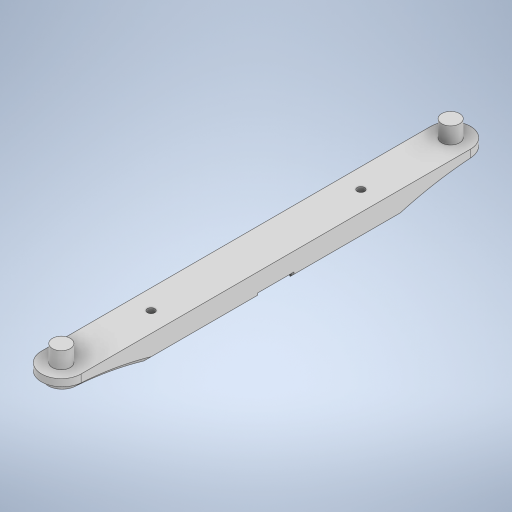
# Autodesk Inventor part: gripper_mechanism
Saved by Autodesk Inventor 2023 (Build 270158000, 158)
## iProperties
Created: 2024-07-03
Part Number: gripper_mechanism
Material: Generic
Document SubType Name: Modeling
Designer: Swoby
Density: 1 g/cm^3
Appearance: Default
Author: Swoby
Autodesk Inventor part; units mm, degrees
ref_plane "YZ Plane" through (0, 0, 0) normal (1, 0, 0) x (0, 1, 0)
ref_plane "XZ Plane" through (0, 0, 0) normal (0, 1, 0) x (-1, 0, 0)
ref_plane "XY Plane" through (0, 0, 0) normal (0, 0, 1) x (1, 0, 0)
sketch "Sketch1" plane through (0, 0, 0) normal (0, 1, 0) x (-1, 0, 0)
  circle A0 centre (0, 29.5) radius 1.5
  circle A1 centre (0, -29.5) radius 1.5
  line L0 (0, 29.5) -> (0, -29.5) construction
  circle A2 centre (0, 29.5) radius 3
  circle A3 centre (0, -29.5) radius 3
  line L1 (3, 29.5) -> (3, -29.5)
  line L2 (-3, 29.5) -> (-3, -29.5)
  point P0 (0, 0)
  dimension "d0" = 59
  dimension "d1" = 29.5
  dimension "d2" = 3
  dimension "d3" = 3
  dimension "d4" = 6
  dimension "d5" = 6
  constraints: 6 end point, 4 centre point, 4 point on circle, 4 tangent, 2 coincident, 1 midpoint, 1 vertical
  measures "d0" distance of L0.end L0.start
  measures "d1" distance of L0.start point (0, 0)
  measures "d2" diameter of A0
  measures "d3" diameter of A1
  measures "d4" diameter of A2
  measures "d5" diameter of A3
extrude "Extrusion1" add sketch "Sketch1" along normal blind 4.05
sketch "Sketch2" plane through (0, 0, 0) normal (0, -1, 0) x (1, 0, 0)
  circle A0 centre (0, 0) radius 3.75
  dimension "d8" = 7.5
  constraints: 1 centre point, 1 coincident
  measures "d8" diameter of A0
extrude "Extrusion2" cut sketch "Sketch2" against normal blind 1.3
sketch "Sketch3" plane through (0, 0, 0) normal (0, -1, 0) x (1, 0, 0)
  circle A0 centre (0, 15.9) radius 0.55
  arc A1 (3, 2.25) -> (-3, 2.25) centre (0, 0) ccw projected
  line L0 (3, 29.5) -> (3, 2.25) projected
  arc A2 (3, 29.5) -> (-3, 29.5) centre (0, 29.5) ccw projected
  line L1 (-3, 2.25) -> (-3, 29.5) projected
  circle A3 centre (0, 29.5) radius 1.5 projected
  arc A4 (-3, -2.25) -> (3, -2.25) centre (0, 0) ccw projected
  line L2 (-3, -29.5) -> (-3, -2.25) projected
  arc A5 (-3, -29.5) -> (3, -29.5) centre (0, -29.5) ccw projected
  line L3 (3, -2.25) -> (3, -29.5) projected
  circle A6 centre (0, -29.5) radius 1.5 projected
  arc A7 (3, 29.5) -> (-3, 29.5) centre (0, 29.5) ccw projected
  line L4 (0, 29.5) -> (0, -29.5)
  circle A8 centre (0, -15.9) radius 0.55
  dimension "d11" = 1.1
  dimension "d12" = 15.9
  dimension "d40" = 1.1
  dimension "d41" = 15.9
  constraints: 2 centre point, 2 end point, 2 point on line, 1 midpoint, 1 vertical
  measures "d11" diameter of A0
  measures "d12" distance of point (0, 0) A0.centre
  measures "d40" diameter of A8
  measures "d41" distance of point (0, 0) A8.centre
extrude "Extrusion3" cut sketch "Sketch3" against normal blind 4.05 contours A0 L4 | L4 A0 | A8 L4 | L4 A8
sketch "Sketch4" plane through (3, 0, -29.5) normal (1, 0, 0) x (0, 0, -1)
  line L0 (-59, 0) -> (-31.75, 0) projected
  line L1 (-62, 0) -> (-62, 4.05) projected
  arc A0 (-48.5, 0) -> (-62, 2) centre (-62.5089, -47.9974) ccw
  line L2 (-62, 2) -> (-62, 0)
  line L3 (-48.5, 0) -> (-62, 0)
  line L4 (3, 2) -> (3, 0)
  line L5 (3, 0) -> (-10.5, 0)
  arc A1 (3, 2) -> (-10.5, 0) centre (3.5089, -47.9974) ccw
  line L6 (3, 0) -> (3, 4.05) projected
  line L7 (-27.25, 1.3) -> (-27.25, 0) projected
  line L8 (-27.25, 0) -> (0, 0) projected
  line L9 (0, 0) -> (0, 4.05) projected
  line L10 (-59, 4.05) -> (0, 4.05) projected
  line L11 (-59, 0) -> (-59, 4.05) projected
  line L12 (-59, 0) -> (-31.75, 0) projected
  line L13 (-31.75, 0) -> (-31.75, 1.3) projected
  line L14 (-31.75, 1.3) -> (-27.25, 1.3) projected
  point P0 (-29.5, 1.3)
  dimension "d18" = 38
  dimension "d19" = 19
  dimension "d20" = 2
  dimension "d21" = 2
  dimension "d22" = 50
  dimension "d23" = 50
  constraints: 8 end point, 5 point on line, 4 point on circle, 2 centre point, 2 collinear, 1 midpoint, 1 perpendicular
  measures "d18" distance of L5.end L3.start
  measures "d19" horizontal distance of L5.end point (-29.5, 1.3)
  measures "d20" distance of L1.start L2.start
  measures "d21" distance of L4.end L4.start
  measures "d22" radius of A0
  measures "d23" radius of A1
extrude "Extrusion4" cut sketch "Sketch4" against normal through all contours L11 A0 L0 | L3 L1 A0 L11 | L9 L5 A1 | A1 L4 L5 L9
chamfer "Chamfer2" distance 1 angle 45 12 edges at (3, 1.2205, 24.1997) (1.9501, 1.9875, 31.7797) (-1.9483, 1.9875, 31.7813) (-3, 1.2205, 24.1997) (3, 0, 10.625) (-3, 0, 10.625) (1.9483, 1.9875, -31.7813) (-1.9501, 1.9875, -31.7797) (-3, 1.2205, -24.1997) (3, 1.2205, -24.1997) (-3, 0, -10.625) (3, 0, -10.625)
chamfer "Chamfer3" distance 0.5 angle 45 4 edges at (-3, 1.15, 2.25) (3, 1.15, 2.25) (-3, 1.15, -2.25) (3, 1.15, -2.25)
sketch "Sketch5" plane through (0, 4.05, 0) normal (0, 1, 0) x (1, 0, 0)
  circle A0 centre (0, -29.5) radius 1.5 projected
  circle A1 centre (0, 29.5) radius 1.5 projected
  point P0 (0, 0)
extrude "Extrusion5" add sketch "Sketch5" against normal blind 2.3
sketch "Sketch6" plane through (0, 1.75, 29.5) normal (0, -1, 0) x (1, 0, 0)
  circle A0 centre (0, 0) radius 1.5 projected
  circle A1 centre (0, -59) radius 1.5 projected
  arc A2 (3, 0) -> (-3, 0) centre (0, 0) ccw projected
  circle A3 centre (0, 0) radius 1.35
  circle A4 centre (0, -59) radius 1.35
  point P0 (0, -29.5)
  dimension "d36" = 2.7
  dimension "d37" = 2.7
  constraints: 2 centre point, 2 coincident
  measures "d36" diameter of A3
  measures "d37" diameter of A4
extrude "Extrusion6" add sketch "Sketch6" against normal blind 4.8 contours A3 | A4
equation "\"d1\" = 0.5 * d0"
equation "\"d40\" = d11"
equation "\"d41\" = d12"
equation "\"d37\" = d36"
body "Solid1"
